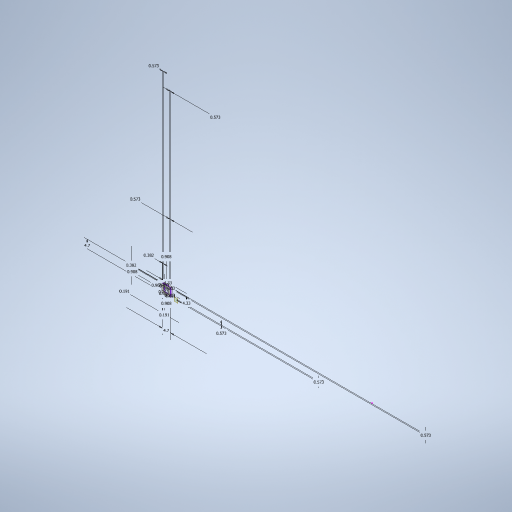
# Autodesk Inventor part: mnt298bracket
Saved by Autodesk Inventor 2024 (Build 280153000, 153)
## iProperties
Created: 2024-04-22
Part Number: mnt298bracket
Material: Generic
Document SubType Name: Modeling
Designer: Ruki
Density: 1 g/cm^3
Appearance: Default
Author: Ruki
Autodesk Inventor part; units mm, degrees
ref_plane "YZ Plane" through (0, 0, 0) normal (1, 0, 0) x (0, 1, 0)
ref_plane "XZ Plane" through (0, 0, 0) normal (0, 1, 0) x (-1, 0, 0)
ref_plane "XY Plane" through (0, 0, 0) normal (0, 0, 1) x (1, 0, 0)
ref_plane "Work Plane3" through (-1117.6, -50.8, 0) normal (0, 0, -1) x (-1, 0, 0)
sketch "Sketch1" plane through (-1117.6, -50.8, 0) normal (0, 0, -1) x (-1, 0, 0)
  line L0 (76.5714, 47.2114) -> (29.5714, 47.2114)
  line L1 (29.5714, 47.2114) -> (29.5714, 0.2114)
  line L2 (29.5714, 0.2114) -> (76.5714, 0.2114)
  line L3 (76.5714, 0.2114) -> (76.5714, 47.2114)
  circle A0 centre (70.838, 41.6003) radius 1.3139
  line L4 (74.6603, 45.4225) -> (31.3603, 45.4225)
  line L5 (31.3603, 45.4225) -> (31.3603, 2.1225)
  line L6 (31.3603, 2.1225) -> (74.6603, 2.1225)
  line L7 (74.6603, 2.1225) -> (74.6603, 45.4225)
  circle A1 centre (35.3047, 41.4781) radius 1.3139
  circle A2 centre (35.3047, 5.9448) radius 1.3139
  circle A3 centre (70.838, 5.9448) radius 1.3139
  circle A4 centre (35.3047, 5.9448) radius 3.1056
  circle A5 centre (70.838, 5.9448) radius 3.1056
  circle A6 centre (70.838, 41.6003) radius 3.1056
  circle A7 centre (35.3047, 41.4781) radius 3.1056
  line L8 (38.6492, 9.2892) -> (67.4936, 9.2892)
  line L9 (67.4936, 9.2892) -> (67.4936, 38.1337)
  line L10 (67.4936, 38.1337) -> (38.6492, 38.1337)
  line L11 (38.6492, 38.1337) -> (38.6492, 9.2892)
  point P0 (-1117.6, 50.8)
  point P1 (53.0714, 47.2114)
  point P2 (53.0714, 0.2114)
  dimension "d1" = 47
  dimension "d2" = 47
  dimension "d4" = 2.6278
  dimension "d5" = 5.7333
  dimension "d6" = 1.9111
  dimension "d7" = 1.9111
  dimension "d8" = 43.3
  dimension "d9" = 43.3
  dimension "d10" = 2.6278
  dimension "d11" = 3.8222
  dimension "d12" = 5.7333
  dimension "d13" = 5.7333
  dimension "d14" = 2.6278
  dimension "d15" = 5.7333
  dimension "d16" = 5.7333
  dimension "d17" = 2.6278
  dimension "d18" = 5.7333
  dimension "d19" = 3.8222
  dimension "d20" = 6.2111
  dimension "d21" = 6.2111
  dimension "d22" = 6.2111
  dimension "d23" = 6.2111
  dimension "d24" = 9.0778
  dimension "d25" = 9.0778
  dimension "d26" = 9.0778
  dimension "d27" = 9.0778
  constraints: 24 end point, 8 centre point, 6 parallel, 4 coincident, 3 horizontal, 3 perpendicular, 2 midpoint
  measures "d1" distance of point (53.071, 47.211) point (53.071, 0.211)
  measures "d2" distance between parallel lines of L1 L3
  measures "d4" diameter of A0
  measures "d5" distance from line of L3 A0.centre
  measures "d6" distance between parallel lines of L3 L7
  measures "d7" distance between parallel lines of L2 L6
  measures "d8" distance between parallel lines of L5 L7
  measures "d9" distance between parallel lines of L6 L4
  measures "d10" diameter of A1
  measures "d11" distance from line of L4 A0.centre
  measures "d12" distance from line of L1 A1.centre
  measures "d13" distance from line of L0 A1.centre
  measures "d14" diameter of A2
  measures "d15" distance from line of L1 A2.centre
  measures "d16" distance from line of L2 A2.centre
  measures "d17" diameter of A3
  measures "d18" distance from line of L2 A3.centre
  measures "d19" distance from line of L7 A3.centre
  measures "d20" diameter of A4
  measures "d21" diameter of A5
  measures "d22" diameter of A6
  measures "d23" diameter of A7
  measures "d24" distance between parallel lines of L1 L11
  measures "d25" distance between parallel lines of L3 L9
  measures "d26" distance between parallel lines of L2 L8
  measures "d27" distance between parallel lines of L0 L10
extrude "Extrusion3" add sketch "Sketch1" along normal blind 8 contours L3 L2 L1 L0
extrude "Extrusion6" add sketch "Sketch1" along normal blind 10 contours A0 | A1 | A2 | A3
extrude "Extrusion7" add sketch "Sketch1" along normal blind 4 contours A2 | A4 | A5 | A6 | A7
extrude "Extrusion8" add sketch "Sketch1" against normal blind 3 contours L3 L2 L1 L0 | A0 | L7 L6 L5 L4 | A1 | A2 | A3 | A4 | A5 | A6 | A7
fillet "Fillet5" radius 10 4 edges at (-1156.2492, -12.6663, 1.5) (-1185.0936, -12.6663, 1.5) (-1185.0936, -41.5108, 1.5) (-1156.2492, -41.5108, 1.5)
fillet "Fillet6" radius 2 4 edges at (-1194.1714, -3.5886, -2.5) (-1147.1714, -3.5886, -2.5) (-1194.1714, -50.5886, -2.5) (-1147.1714, -50.5886, -2.5)
body "Solid2"
